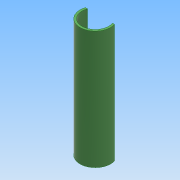
# Autodesk Inventor part: Top_Tilt Pipe_3 Lanes
Saved by Autodesk Inventor 2018.1 (Build 221171000, 171)
## iProperties
Created: 2019-02-25
Part Number: Top_Tilt Pipe_3 Lanes
Material: PVC-Piping
Document SubType Name: Modeling
Designer: James
Density: 1.4 g/cm^3
Appearance: Smooth - Dark Forest Green
Author: James
Autodesk Inventor part; units mm, degrees
ref_plane "YZ Plane" through (0, 0, 0) normal (1, 0, 0) x (0, 1, 0)
ref_plane "XZ Plane" through (0, 0, 0) normal (0, 1, 0) x (-1, 0, 0)
ref_plane "XY Plane" through (0, 0, 0) normal (0, 0, 1) x (1, 0, 0)
sketch "Sketch1" plane through (0, 0, 0) normal (0, 0, 1) x (1, 0, 0)
  circle A0 centre (0, 0) radius 20
  circle A1 centre (0, 0) radius 23
  dimension "d0" = 40
  dimension "d1" = 46
  constraints: 2 centre point, 2 coincident
  measures "d0" diameter of A0
  measures "d1" diameter of A1
extrude "Extrusion1" add sketch "Sketch1" along normal mid plane 178
sketch "Sketch2" plane through (0, 0, 0) normal (1, 0, 0) x (0, 1, 0)
  line L0 (0, 70) -> (0, -70) projected
  line L1 (-70, 0) -> (70, 0) projected
  point P0 (0, 0)
  point P1 (0, 35)
  point P2 (0, -35)
  dimension "d19" = 35
  dimension "d20" = 70
  measures "d19" distance of point (0, 35) point (0, 0)
  measures "d20" distance of point (0, 35) point (0, -35)
hole "Hole1" at (0, 0, 35) at (0, 0, -35) direction (-1, 0, 0) diameter 4.5 end through all clearance for "Flat Head Machine Screw" size "M4" standard "Ansi Metric M Profile"
sketch "Sketch3" plane through (0, 0, 0) normal (1, 0, 0) x (0, 1, 0)
  line L0 (23, -89) -> (7, -89)
  line L1 (7, -89) -> (7, 89)
  line L2 (7, 89) -> (23, 89)
  line L3 (23, 89) -> (23, -89)
  line L4 (23, 89) -> (-23, 89) projected
  line L5 (-23, -89) -> (23, -89) projected
  line L6 (0, 159.6) -> (0, -159.6) projected
  point P0 (0, 0)
  dimension "d13" = 0
  dimension "d14" = 0
  dimension "d15" = 7
  constraints: 8 end point, 2 parallel, 1 coincident, 1 horizontal, 1 perpendicular
  measures "d13" distance between parallel lines of L4 L2
  measures "d14" distance between parallel lines of L5 L0
  measures "d15" distance between parallel lines of L6 L1
extrude "Extrusion2" cut sketch "Sketch3" along normal through all both and the other way through all contours L0 L1 L2 L3
equation "\"d19\" = 0.5 * d20"
body "Solid1"
